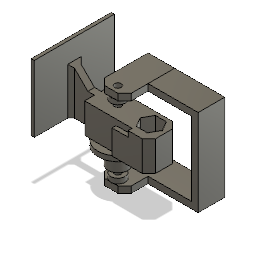
7Segment-Klappanzeige Klappelement v6 (Autodesk Fusion 360 design; units mm, degrees)
Autodesk Fusion 360 part; units mm, degrees
sketch "Skizze1" plane through (0, 0, 0) normal (0, 1, 0) x (1, 0, 0)
  circle A0 centre (0, 0) radius 1
  circle A1 centre (0, 0) radius 2.3
  line L0 (-14, 7) -> (-14, -5) construction
  line L1 (0, 0) -> (-16, 0) construction
  line L2 (-6, 3.95) -> (14.4, 3.95)
  line L3 (14.4, 3.95) -> (14.4, -3.95)
  line L4 (14.4, -3.95) -> (-6, -3.95)
  line L5 (-6, -3.95) -> (-6, 3.95)
  line L6 (-14, 12) -> (-13, 12)
  line L7 (-13, 12) -> (-13, -12)
  line L8 (-13, -12) -> (-14, -12)
  line L9 (-14, -12) -> (-14, 12)
  line L10 (-13, 1) -> (-6, 1)
  line L11 (-6, 1) -> (-6, -1)
  line L12 (-6, -1) -> (-13, -1)
  line L13 (-13, -1) -> (-13, 1)
  line L14 (14.4, -3.95) -> (3.4, -3.95)
  line L15 (3.4, -3.95) -> (3.4, -5.15)
  line L16 (3.4, -5.15) -> (14.4, -5.15)
  line L17 (14.4, -5.15) -> (14.4, -3.95)
  line L18 (8.2, -5.15) -> (8.2, -3.95)
  line L19 (13.2909, 0) -> (11.6454, 2.85)
  line L20 (11.6454, 2.85) -> (8.3546, 2.85)
  line L21 (8.3546, 2.85) -> (6.7091, 0)
  line L22 (6.7091, 0) -> (8.3546, -2.85)
  line L23 (8.3546, -2.85) -> (11.6454, -2.85)
  line L24 (11.6454, -2.85) -> (13.2909, 0)
  point P0 (10, 0)
  dimension "d1" = 2
  dimension "d2" = 4.6
  dimension "d3" = 14
  dimension "d4" = 7.9
  dimension "d5" = 1
  dimension "d6" = 2
  dimension "d7" = 6
  dimension "d8" = 14.4
  dimension "d9" = 11
  dimension "d10" = 1.2
  dimension "d11" = 4.8
  dimension "d12" = 24
  dimension "d57" = 5.7
  dimension "d58" = 10
  constraint coincident A0.centre A1.centre
  constraint vertical L0
  constraint perpendicular L0 L1
  constraint horizontal L2
  constraint vertical L3
  constraint horizontal L4
  constraint vertical L5
  constraint symmetric L1 L2 L4
  constraint horizontal L6
  constraint vertical L7
  constraint horizontal L8
  constraint vertical L9
  constraint coincident L0 L6.start
  constraint horizontal L10
  constraint vertical L11
  constraint horizontal L12
  constraint vertical L13
  constraint coincident L5 L11.end
  constraint coincident L7 L10.start
  constraint symmetric L1 L10 L12
  constraint symmetric L1 L6 L8
  constraint horizontal L14
  constraint vertical L15
  constraint horizontal L16
  constraint vertical L17
  constraint coincident L16 L18.start
  constraint perpendicular L16 L18
  constraint coincident L4 L18.end
  constraint horizontal L20
  constraint coincident L1 P0
  measures "d1" diameter of A0
  measures "d2" diameter of A1
  measures "d3" distance of A0.centre L0
  measures "d4" distance of L2 L4
  measures "d5" distance of L6.start L6.end
  measures "d6" distance of L10 L12
  measures "d7" distance of A0.centre L5
  measures "d8" distance of A0.centre L3
  measures "d9" distance of L15.end L16.end
  measures "d10" distance of L3.end L16.end
  measures "d11" distance of L15 L18
  measures "d12" distance of L6.start L8.end
  measures "d57" distance of L20 L23
  measures "d58" distance of A0.centre P0
extrude "Extrusion1" add sketch "Skizze1" along normal blind 9 contours A1 | L2 L3 L4 L5 L11 L14 | L5 L7 L10 L11 L12 L13 | L4 L14 L16 L17 L18 | L6 L7 L8 L9 L13 makes body 1
extrude "Extrusion2" add sketch "Skizze1" along normal blind 7.3 contours L4 L14 L15 L16 L18 bodies 1
extrude "Extrusion4" add sketch "Skizze1" along normal blind 20 contours L6 L7 L8 L9 L13 bodies 1
chamfer "Fase3" distance 2 angle 45 2 edges at (14.4, 4.5, 5.15) (14.4, 4.5, -3.95) on bodies 1
chamfer "Fase2" distance 5 angle 45 1 edges at (-13, 9, 0) on bodies 1
chamfer "Chamfer5" distance 1 angle 45 2 edges at (-13, 7, 1) (-13, 7, -1) on bodies 1
extrude "Extrude12" add sketch "Skizze1" along normal blind 1 contours L19 L20 L21 L22 L23 L24 bodies 1
sketch "Skizze2" plane through (0, 0, 0) normal (0, 1, 0) x (1, 0, 0)
  circle A0 centre (0, 0) radius 1
  circle A1 centre (0, 0) radius 3
  circle A2 centre (0, 0) radius 6
  dimension "d23" = 6
  dimension "d24" = 12
  constraint concentric A0 A1
  constraint concentric A1 A2
  constraint coincident A0.centre A1.centre
  measures "d23" diameter of A1
  measures "d24" diameter of A2
extrude "Extrusion5" add sketch "Skizze2" against normal blind 1.5 separate body contours A1 | A2 makes body 2
extrude "Extrusion6" add sketch "Skizze2" against normal blind 5.5 from surface at -1 contours A1 bodies 2
sketch "Skizze3" plane through (0, 0, 0) normal (0, 0, 1) x (1, 0, 0)
  line L0 (-4, 12) -> (4, 12)
  line L1 (4, 12) -> (4, 14)
  line L2 (4, 14) -> (-4, 14)
  line L3 (-4, 14) -> (-4, 12)
  line L4 (-4, -10) -> (4, -10)
  line L5 (4, -10) -> (4, -12)
  line L6 (4, -12) -> (-4, -12)
  line L7 (-4, -12) -> (-4, -10)
  line L8 (0, 1.75) -> (0, 22.5)
  line L9 (4, -12) -> (19, -12)
  line L10 (19, -12) -> (19, 14)
  line L11 (19, 14) -> (4, 14)
  line L12 (4, 12) -> (17, 12)
  line L13 (17, 12) -> (17, -10)
  line L14 (17, -10) -> (4, -10)
  dimension "d31" = 8
  dimension "d33" = 2
  dimension "d34" = 2
  dimension "d35" = 22
  dimension "d36" = 12
  dimension "d37" = 2
  dimension "d38" = 13
  constraint horizontal L0
  constraint vertical L1
  constraint horizontal L2
  constraint vertical L3
  constraint horizontal L4
  constraint vertical L5
  constraint horizontal L6
  constraint vertical L7
  constraint symmetric L1 L3 L8
  constraint symmetric L5 L7 L8
  constraint collinear L1 L5
  constraint perpendicular L5 L9
  constraint perpendicular L9 L10
  constraint perpendicular L1 L12
  constraint perpendicular L0 L13
  constraint horizontal L14
  constraint horizontal L11
  measures "d31" distance of L5.end L6.end
  measures "d33" distance of L0.end L1.end
  measures "d34" distance of L4.end L5.end
  measures "d35" distance of L0 L4
  measures "d36" distance of origin L0
  measures "d37" distance of L10 L13
  measures "d38" distance of L4.end L13.end
extrude "Extrusion7" add sketch "Skizze3" along normal blind -5 and the other way blind -2 separate body contours L0 L2 L3 L8 | L0 L1 L2 L8 | L4 L5 L6 L7 makes body 3 at (1.3333, -12, -0.3333) makes body 4 at (-1.3333, 12, -0.3333)
extrude "Extrusion8" add sketch "Skizze3" against normal blind 8 from surface at -5 bodies 3 4
sketch "Skizze4" plane through (0, -10, 0) normal (0, 1, 0) x (-1, 0, 0)
  line L0 (4, 2) -> (-4, 2)
  line L1 (-4, 2) -> (-4, -5)
  line L2 (-4, -5) -> (-17, -5)
  line L3 (-17, -5) -> (-17, -13)
  line L4 (-17, -13) -> (4, -13)
  line L5 (4, -13) -> (4, 2)
  circle A0 centre (0, 0) radius 1
  circle A1 centre (0, 0) radius 2.15
  dimension "d44" = 2
  dimension "d45" = 4.3
  constraint coincident A0.centre A1.centre
  constraint concentric A0 A1
  measures "d44" diameter of A0
  measures "d45" diameter of A1
extrude "Extrusion9" add sketch "Skizze4" along normal blind 1.5 contours L0 A1 | L0 A1 bodies 3
extrude "Extrusion10" add sketch "Skizze4" against normal blind 1.5 from surface at 22 contours L0 A1 | L0 A1 bodies 3
extrude "Extrusion11" cut sketch "Skizze4" along normal through all and the other way through all contours A0 bodies 3
chamfer "Fase4" distance 2 angle 45 4 edges at (4, 13, 2) (-4, 13, 2) (-4, -11, 2) (4, -11, 2) on bodies 3
named bodies: "Klappelement", "MagnetHalter", "Wellenlager"
